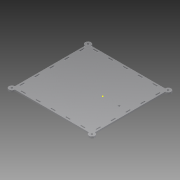
# Autodesk Inventor part: BasePlate2
Saved by Autodesk Inventor 2015 SP1 (Build 190203100, 203)
## iProperties
Created: 2014-08-06
Part Number: BasePlate2
Material: Acrylic, Clear
Document SubType Name: Modeling
Designer: Patrick Camilleri
Density: 1.19 g/cm^3
Appearance: Transparent - Clear
Mass: 654.149 g
Surface Area: 1962.87 cm^2
Volume: 549.705 cm^3
Author: Patrick Camilleri
Autodesk Inventor part; units mm, degrees
ref_plane "YZ Plane" through (0, 0, 0) normal (1, 0, 0) x (0, 1, 0)
ref_plane "XZ Plane" through (0, 0, 0) normal (0, 1, 0) x (-1, 0, 0)
sketch "Sketch1" plane through (0, 0, 0) normal (0, 0, 1) x (1, 0, 0)
  line L0 (-177, -128) -> (92, -128)
  line L1 (92, -128) -> (92, 128)
  line L2 (92, 128) -> (-177, 128)
  line L3 (-177, 128) -> (-177, -128)
  line L4 (-177, 0) -> (92, 0) construction
  line L5 (0, -128) -> (0, 128) construction
  point P0 (0, 0)
  point P1 (0, 0)
  dimension "d160" = 256
  dimension "d161" = 177
  dimension "d162" = 92
  constraints: 12 end point, 3 midpoint, 2 parallel, 2 perpendicular, 2 point on line, 1 coincident, 1 horizontal
  measures "d160" distance of L0.end L1.end
  measures "d161" distance between parallel lines of L3 L5
  measures "d162" distance between parallel lines of L1 L5
extrude "Extrusion1" add sketch "Sketch1" along normal blind 5
sketch "Sketch2" plane through (0, 0, 5) normal (0, 0, 1) x (1, 0, 0)
  line L0 (-172.1, 7.475) -> (-168.9, 7.475)
  line L1 (-168.9, 7.475) -> (-168.9, -7.475)
  line L2 (-168.9, -7.475) -> (-172.1, -7.475)
  line L3 (-172.1, -7.475) -> (-172.1, 7.475)
  line L4 (-172.1, 7.475) -> (-168.9, -7.475) construction
  line L5 (-168.9, 7.475) -> (-172.1, -7.475) construction
  line L6 (-177, -128) -> (92, -128) projected
  line L7 (92, -128) -> (92, 128) projected
  line L8 (92, 128) -> (-177, 128) projected
  line L9 (-177, 128) -> (-177, -128) projected
  line L10 (83.9, -7.475) -> (87.1, -7.475)
  line L11 (87.1, -7.475) -> (87.1, 7.475)
  line L12 (87.1, 7.475) -> (83.9, 7.475)
  line L13 (83.9, 7.475) -> (83.9, -7.475)
  line L14 (83.9, -7.475) -> (87.1, 7.475) construction
  line L15 (87.1, -7.475) -> (83.9, 7.475) construction
  line L16 (-170.5, -121.5) -> (85.5, -121.5) construction
  line L17 (85.5, -121.5) -> (85.5, 121.5) construction
  line L18 (85.5, 121.5) -> (-170.5, 121.5) construction
  line L19 (-170.5, 121.5) -> (-170.5, -121.5) construction
  point P0 (0, 0)
  point P1 (-170.5, 0)
  point P2 (85.5, 0)
  point P3 (85.5, 0)
  point P4 (-170.5, 0)
  dimension "d77" = 3.2
  dimension "d78" = 14.95
  dimension "d163" = 3.2
  dimension "d164" = 14.95
  dimension "d187" = 6.5
  constraints: 32 end point, 8 midpoint, 4 parallel, 2 horizontal, 2 perpendicular, 3 other
  measures "d77" distance of L1.end L2.end
  measures "d78" distance of L0.end L1.end
  measures "d163" distance of L12.end L11.end
  measures "d164" distance of L11.end L10.end
  measures "d187" distance between parallel lines of L9 L19
extrude "Extrusion3" cut sketch "Sketch2" against normal through all contours L0 L1 L2 L3 | L13 L12 L11 L10
sketch "Sketch3" plane through (0, 0, 5) normal (0, 0, 1) x (1, 0, 0)
  line L0 (-152.475, 123.1) -> (-137.525, 123.1)
  line L1 (-137.525, 123.1) -> (-137.525, 119.9)
  line L2 (-137.525, 119.9) -> (-152.475, 119.9)
  line L3 (-152.475, 119.9) -> (-152.475, 123.1)
  line L4 (-152.475, 123.1) -> (-137.525, 119.9) construction
  line L5 (-137.525, 123.1) -> (-152.475, 119.9) construction
  line L6 (-152.475, -119.9) -> (-137.525, -119.9)
  line L7 (-137.525, -119.9) -> (-137.525, -123.1)
  line L8 (-137.525, -123.1) -> (-152.475, -123.1)
  line L9 (-152.475, -123.1) -> (-152.475, -119.9)
  line L10 (-152.475, -119.9) -> (-137.525, -123.1) construction
  line L11 (-137.525, -119.9) -> (-152.475, -123.1) construction
  line L12 (-172.1, -7.475) -> (-172.1, 7.475) projected
  line L13 (-172.1, 7.475) -> (-168.9, 7.475) projected
  line L14 (-168.9, 7.475) -> (-168.9, -7.475) projected
  line L15 (-168.9, -7.475) -> (-172.1, -7.475) projected
  line L16 (-177, -128) -> (92, -128) projected
  line L17 (92, 128) -> (-177, 128) projected
  line L18 (-177, 128) -> (-177, -128) projected
  point P0 (0, 0)
  point P1 (-145, 121.5)
  point P2 (-145, -121.5)
  dimension "d125" = 14.95
  dimension "d126" = 3.2
  dimension "d128" = 14.95
  dimension "d129" = 3.2
  dimension "d198" = 32
  dimension "d199" = 6.5
  dimension "d200" = 32
  dimension "d201" = 6.5
  constraints: 24 end point, 4 midpoint, 4 parallel, 2 horizontal, 2 perpendicular
  measures "d125" distance of L1.end L2.end
  measures "d126" distance of L0.end L1.end
  measures "d128" distance of L7.end L8.end
  measures "d129" distance of L6.end L7.end
  measures "d198" distance from line of L18 point (-145, 121.5)
  measures "d199" distance from line of L17 point (-145, 121.5)
  measures "d200" distance from line of L18 point (-145, -121.5)
  measures "d201" distance from line of L16 point (-145, -121.5)
extrude "Extrusion4" cut sketch "Sketch3" against normal through all contours L0 L1 L2 L3 | L6 L7 L8 L9
pattern_linear "Rectangular Pattern1" count 5 spacing 50 along (1, 0, 0) of "Extrusion4"
pattern_linear "Rectangular Pattern2" count 5 spacing 50 along (0, -1, 0) of "Extrusion3" first direction both ways yes
sketch "Sketch7" plane through (0, 0, 5) normal (0, 0, 1) x (1, 0, 0)
  circle A0 centre (-177, -128) radius 10
  circle A1 centre (92, -128) radius 10
  point P0 (0, 0)
  dimension "d165" = 20
  dimension "d166" = 20
  constraints: 2 centre point, 2 coincident
  measures "d165" diameter of A0
  measures "d166" diameter of A1
extrude "Extrusion6" add sketch "Sketch7" against normal blind 6
mirror "Mirror7" about plane through (0, 0, 0) normal (0, 1, 0) of "Extrusion6"
hole "Hole6" at (-177, -128, 5) direction (0, 0, -1) diameter 6 end through all
hole "Hole7" at (92, -128, 5) direction (0, 0, -1) diameter 6 end through all
mirror "Mirror8" about plane through (0, 0, 0) normal (0, 1, 0) of "Hole6", "Hole7"
sketch "Sketch9" plane through (0, 0, 5) normal (0, 0, 1) x (1, 0, 0)
  line L0 (-168.9, 7.475) -> (-168.9, -7.475) projected
  line L1 (53.25, 2.425) -> (58.2, 2.425)
  line L2 (58.2, 2.425) -> (58.2, -2.425)
  line L3 (58.2, -2.425) -> (53.25, -2.425)
  line L4 (53.25, -2.425) -> (53.25, 2.425)
  point P0 (0, 0)
  point P1 (53.25, 0)
  point P2 (53.25, 0)
  dimension "d193" = 222.15
  dimension "d194" = 4.95
  dimension "d195" = 4.85
  constraints: 8 end point, 2 parallel, 1 coincident, 1 horizontal, 1 midpoint, 1 perpendicular
  measures "d193" distance from line of point (53.25, 0) L0
  measures "d194" distance of L2.end L3.end
  measures "d195" distance of L1.end L2.end
extrude "Extrusion8" cut sketch "Sketch9" against normal through all
sketch "Sketch11" plane through (0, 0, 5) normal (0, 0, 1) x (1, 0, 0)
  point P0 (0, 0)
ref_plane "Work Plane1" through (0, 0, 5) normal (0, 1, 0) x (1, 0, 0)
sketch "Sketch13" plane through (0, 0, 5) normal (0, 0, 1) x (1, 0, 0)
  point P0 (0, 0)
equation "\"d166\" = d165"
equation "\"kerf\" = 0.15"
equation "\"slot_w\" = 3.35"
equation "\"slot_l\" = 15.1"
body "Solid1"
